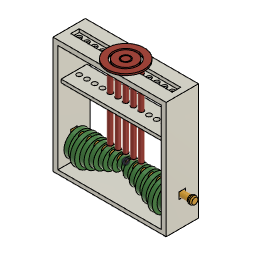
water-drop-mech (Autodesk Fusion 360 design; units mm, degrees)
Autodesk Fusion 360 part; units mm, degrees
note: some values were not read from the file. Set by a fixed rule: which face or edge a step refers to.
sketch "holder body" plane through (0, 0, 0) normal (0, 1, 0) x (1, 0, 0) in component "holder"
  line L0 (107, -220) -> (-68, -220)
  line L1 (-68, -220) -> (-68, -40)
  line L2 (-68, -40) -> (107, -40)
  line L3 (107, -40) -> (107, -220)
  line L4 (107, -220) -> (97, -220)
  line L5 (107, -210) -> (107, -220)
  line L6 (-68, -40) -> (-58, -40)
  line L7 (-68, -50) -> (-68, -40)
  line L8 (97, -210) -> (97, -170)
  line L9 (107, -170) -> (107, -210)
  line L10 (97, -170) -> (-58, -170)
  line L11 (-68, -170) -> (-68, -160)
  line L12 (-58, -160) -> (97, -160)
  line L13 (107, -160) -> (107, -170)
  line L14 (97, -210) -> (-68, -210)
  line L15 (-68, -210) -> (-68, -220)
  line L16 (-68, -220) -> (97, -220)
  line L17 (-68, -50) -> (-68, -210)
  line L18 (-58, -210) -> (-58, -50)
  line L19 (-58, -50) -> (97, -50)
  line L20 (107, -50) -> (107, -40)
  line L21 (107, -40) -> (-58, -40)
  line L22 (107, -170) -> (107, -50)
  line L23 (97, -50) -> (97, -170)
  dimension "d1" = 175
  dimension "d2" = 180
  dimension "d3" = 10
  dimension "d4" = 10
  dimension "d5" = 10
  dimension "d6" = 10
  dimension "d7" = 10
  dimension "d8" = 175
  dimension "d9" = 10
  constraint horizontal L0
  constraint vertical L1
  constraint horizontal L2
  constraint vertical L3
  constraint horizontal L4
  constraint vertical L5
  constraint horizontal L6
  constraint vertical L7
  constraint vertical L8
  constraint vertical L9
  constraint horizontal L10
  constraint vertical L11
  constraint horizontal L12
  constraint vertical L13
  constraint horizontal L14
  constraint vertical L15
  constraint horizontal L16
  constraint vertical L17
  constraint vertical L18
  constraint horizontal L19
  constraint vertical L20
  constraint horizontal L21
  constraint vertical L22
  constraint vertical L23
  constraint coincident L23 L12.end
  constraint coincident L18 L10.end
  constraint coincident L18 L12.start
  measures "d1" distance of L0.start L0.end
  measures "d2" distance of L0.start L2.end
  measures "d3" distance of L0.start L4.end
  measures "d4" distance of L0.start L5.start
  measures "d5" distance of L1.end L6.end
  measures "d6" distance of L1.end L7.start
  measures "d7" distance of L5.start L8.start
  measures "d8" distance of L9.start L11.start
  measures "d9" distance of L9.start L13.start
extrude "Extrude1" add sketch "holder body" against normal blind 50 makes body 1 in component "holder"
sketch "holder top holes" plane through (0, 0, 220) normal (0, 0, 1) x (-1, 0, 0) in component "holder"
  line L0 (-107, 0) -> (68, 0)
  line L1 (68, 0) -> (68, 50)
  line L2 (68, 50) -> (-107, 50)
  line L3 (-107, 50) -> (-107, 0)
  circle A0 centre (-19.5, 25) radius 3.75
  circle A1 centre (-31.5, 25) radius 3.75
  circle A2 centre (-43.5, 25) radius 3.75
  circle A3 centre (-55.5, 25) radius 3.75
  circle A4 centre (-67.5, 25) radius 3.75
  circle A5 centre (-79.5, 25) radius 3.75
  circle A6 centre (-91.5, 25) radius 3.75
  line L4 (-71.25, 25) -> (-75.75, 25)
  line L5 (-83.25, 25) -> (-87.75, 25)
  line L6 (-95.25, 25) -> (-107, 25)
  line L7 (-59.25, 25) -> (-63.75, 25)
  line L8 (-47.25, 25) -> (-51.75, 25)
  line L9 (-35.25, 25) -> (-39.75, 25)
  line L10 (-23.25, 25) -> (-27.75, 25)
  line L11 (-19.5, 0) -> (-19.5, 21.25)
  line L12 (-19.5, 28.75) -> (-19.5, 50)
  circle A7 centre (-7.5, 25) radius 3.75
  circle A8 centre (4.5, 25) radius 3.75
  circle A9 centre (16.5, 25) radius 3.75
  circle A10 centre (28.5, 25) radius 3.75
  circle A11 centre (40.5, 25) radius 3.75
  circle A12 centre (52.5, 25) radius 3.75
  line L13 (52.5, 25) -> (59, 25)
  line L14 (59, 25) -> (59, 18.5)
  line L15 (-91.5, 25) -> (-98, 25)
  line L16 (-98, 25) -> (-98, 31.5)
  line L17 (-98, 31.5) -> (59, 31.5)
  line L18 (59, 31.5) -> (59, 18.5)
  line L19 (59, 18.5) -> (-98, 18.5)
  line L20 (-98, 18.5) -> (-98, 31.5)
  dimension "d12" = 7.5
  dimension "d15" = 72
  dimension "d16" = 0
  dimension "d19" = 6.5
  dimension "d20" = 6.5
  dimension "d21" = 6.5
  constraint midpoint L3 L6.end
  constraint midpoint L0 L11.start
  constraint perpendicular L0 L11
  constraint coincident A4 L7.end
  constraint coincident A4 L4.start
  constraint coincident A5 L4.end
  constraint coincident A5 L5.start
  constraint collinear L4 L5
  constraint coincident A6 L5.end
  constraint coincident A6 L6.start
  constraint collinear L5 L6
  constraint coincident A3 L8.end
  constraint coincident A3 L7.start
  constraint coincident A2 L9.end
  constraint coincident A2 L8.start
  constraint coincident A1 L10.end
  constraint coincident A1 L9.start
  constraint coincident A0 L10.start
  constraint coincident A0 L11.end
  constraint coincident A0 L12.start
  constraint collinear L11 L12
  constraint symmetric A1 L11 A7
  constraint symmetric A2 L11 A8
  constraint symmetric A3 L11 A9
  constraint symmetric A4 L11 A10
  constraint symmetric A5 L11 A11
  constraint symmetric A6 L11 A12
  constraint coincident A12.centre L13.start
  constraint horizontal L13
  constraint perpendicular L13 L14
  constraint coincident A6.centre L15.start
  constraint parallel L6 L15
  constraint perpendicular L6 L16
  constraint horizontal L17
  constraint vertical L18
  constraint horizontal L19
  constraint vertical L20
  measures "d12" diameter of A0
  measures "d19" distance of L13.end L14.end
  measures "d20" distance of A6.centre L15.end
  measures "d21" distance of L15.end L16.end
extrude "Extrude3" cut sketch "holder top holes" against normal blind 5 contours A0 A1 A2 A3 A4 A5 A6 L4 L5 L6 L7 L8 L9 L10 L11 L15 L19 L20 | A0 L11 L12 L14 L17 L18 L19 | A0 A1 A2 A3 A4 A5 A6 L4 L5 L6 L7 L8 L9 L10 L12 L15 L16 L17 L20 bodies 1 in component "holder"
extrude "Extrude2" cut sketch "holder top holes" against normal blind 44 contours A0 | A6 | A1 | A5 | A2 | A4 | A3 | A7 | A8 | A9 | A10 | A11 | A12 bodies 1 in component "holder"
move_face "OffsetFaces1" offset -0.03 13 faces at (-44.2314, -24.6266, 213.3333) (-56.2314, -24.6266, 213.3333) (-32.2314, -24.6266, 213.3333) (-20.2314, -24.6266, 213.3333) (-8.2314, -24.6266, 213.3333) (3.7686, -24.6266, 213.3333) (15.7686, -25.3734, 213.3333) (27.7686, -25.3734, 213.3333) (39.7686, -25.3734, 213.3333) (51.7686, -25.3734, 213.3333) (63.7686, -25.3734, 213.3333) (75.7686, -25.3734, 213.3333) (87.7686, -25.3734, 213.3333) on bodies 1 in component "holder"
sketch "holder side details" plane through (107, 0, 0) normal (1, 0, 0) x (0, 1, 0) in component "holder"
  line L0 (0, 40) -> (0, 220)
  line L1 (-50, 220) -> (-50, 40)
  line L2 (-50, 40) -> (0, 40)
  line L3 (-50, 40) -> (0, 40)
  line L4 (0, 40) -> (0, 220)
  line L5 (0, 220) -> (-50, 220)
  line L6 (-50, 220) -> (-50, 40)
  line L7 (-25, 40) -> (-25, 220)
  line L8 (-25, 220) -> (-25, 160)
  line L9 (-25, 40) -> (-25, 85)
  line L10 (-20, 80) -> (-30, 80)
  line L11 (-30, 80) -> (-30, 90)
  line L12 (-30, 90) -> (-20, 90)
  line L13 (-20, 90) -> (-20, 80)
  line L14 (-20, 80) -> (-30, 90) construction
  line L15 (-30, 80) -> (-20, 90) construction
  line L16 (-5, 155) -> (-45, 155)
  line L17 (-45, 155) -> (-45, 165)
  line L18 (-45, 165) -> (-5, 165)
  line L19 (-5, 165) -> (-5, 155)
  line L20 (-5, 155) -> (-45, 165) construction
  line L21 (-45, 155) -> (-5, 165) construction
  line L22 (0, 220) -> (-50, 220)
  point P0 (-25, 85)
  point P1 (-25, 160)
  dimension "d26" = 60
  dimension "d27" = 45
  constraint horizontal L3
  constraint vertical L4
  constraint horizontal L5
  constraint vertical L6
  constraint coincident L0.end L4.end
  constraint coincident L1.end L2.start
  constraint midpoint L3 L7.start
  constraint midpoint L5 L7.end
  constraint perpendicular L5 L8
  constraint perpendicular L3 L9
  constraint horizontal L10
  constraint perpendicular L10 L11
  constraint parallel L10 L12
  constraint parallel L11 L13
  constraint coincident L14 P0
  constraint coincident L15 P0
  constraint coincident P0 L9.end
  constraint horizontal L16
  constraint perpendicular L16 L17
  constraint parallel L16 L18
  constraint parallel L17 L19
  constraint coincident L20 P1
  constraint coincident L21 P1
  constraint coincident P1 L8.end
  measures "d26" distance of L7.end P1
  measures "d27" distance of L7.start P0
extrude "Extrude4" cut sketch "holder side details" against normal blind 260 contours L7 L9 L10 L11 L12 | L7 L9 L10 L12 L13 bodies 1 in component "holder"
extrude "Extrude5" add sketch "holder side details" against normal blind 165 contours L7 L8 L16 L18 L19 | L7 L8 L16 L17 L18 bodies 1 in component "holder"
extrude "Extrude6" cut sketch "holder top holes" against normal blind 125 contours A0 | A6 | A1 | A5 | A2 | A4 | A3 | A7 | A8 | A9 | A10 | A11 | A12 bodies 1 in component "holder"
move_face "OffsetFaces2" offset -0.03 13 faces at (75.7686, -24.6266, 161.6667) (87.7686, -24.6266, 161.6667) (63.7686, -24.6266, 161.6667) (51.7686, -24.6266, 161.6667) (39.7686, -24.6266, 161.6667) (27.7686, -24.6266, 161.6667) (15.7686, -24.6266, 161.6667) (3.7686, -24.6266, 161.6667) (-8.2314, -24.6266, 161.6667) (-20.2314, -24.6266, 161.6667) (-32.2314, -24.6266, 161.6667) (-44.2314, -24.6266, 161.6667) (-56.2314, -24.6266, 161.6667) on bodies 1 in component "holder"
extrude "Extrude7" cut 1 faces at (97, -23.3333, 133.3333) along direction (1, 0, 0) blind 2.5 on bodies 1 bodies 1 in component "holder"
extrude "Extrude8" cut 1 faces at (-58, -23.3333, 133.3333) along direction (-1, 0, 0) blind 2.5 on bodies 1 bodies 1 in component "holder"
sketch "support rod" plane through (0, 0, 0) normal (1, 0, 0) x (0, 1, 0) in component "support rod"
  circle A0 centre (0, 0) radius 5
  dimension "d40" = 10
  constraint coincident A0.centre origin
  measures "d40" diameter of A0
extrude "Extrude1'" add sketch "support rod" along normal blind 100 and the other way blind 100 separate body makes body 2 in component "support rod"
move_face "OffsetFaces1'" offset -0.2 2 faces at (33.3333, 4.9752, -0.4978) (-33.3333, 4.9752, -0.4978) on bodies 2 in component "support rod"
extrude "Extrude2'" add 1 faces at (100, 1.1814, 0.0314) along direction (1, 0, 0) blind 2.5 draft 25 on bodies 2 bodies 2 in component "support rod"
extrude "Extrude3'" add 1 faces at (102.5, 1.4577, 1.3526) along direction (1, 0, 0) blind 2 on bodies 2 bodies 2 in component "support rod"
extrude "Extrude4'" add 1 faces at (104.5, 1.4577, 1.3526) along direction (1, 0, 0) blind 2.5 draft -25 on bodies 2 bodies 2 in component "support rod"
sketch "support circle 1" plane through (0, 0, 0) normal (1, 0, 0) x (0, 1, 0) in component "support circle 1"
  circle A0 centre (30, 20) radius 10
  circle A1 centre (30, 22) radius 5
  dimension "d52" = 10
  measures "d52" diameter of A1
extrude "Extrude1''" add sketch "support circle 1" against normal blind 7 separate body makes body 3 in component "support circle 1"
sketch "support circle 2" plane through (0, 0, 0) normal (1, 0, 0) x (0, 1, 0) in component "support circle 2"
  circle A0 centre (0, 0) radius 12.5
  circle A1 centre (0, 5) radius 5
  dimension "d55" = 25
  constraint coincident A0.centre origin
  constraint coincident A0.centre A1
  measures "d55" diameter of A0
extrude "Extrude1'''" add sketch "support circle 2" along normal blind 7 separate body makes body 4 in component "support circle 2"
sketch "support circle 3" plane through (0, 0, 0) normal (1, 0, 0) x (0, 1, 0) in component "support circle 3"
  circle A0 centre (0, 0) radius 15
  circle A1 centre (0, 7.5) radius 5
  constraint coincident A0.centre origin
extrude "Extrude1''''" add sketch "support circle 3" against normal blind 7 separate body makes body 5 in component "support circle 3"
sketch "support circle 4" plane through (0, 0, 0) normal (1, 0, 0) x (0, 1, 0) in component "support circle 4"
  circle A0 centre (0, 0) radius 17.5
  circle A1 centre (0, 10) radius 5
  dimension "d60" = 35
  constraint coincident A0.centre origin
  measures "d60" diameter of A0
extrude "Extrude1'''''" add sketch "support circle 4" along normal blind 7 separate body makes body 6 in component "support circle 4"
sketch "support circle 5" plane through (0, 0, 0) normal (1, 0, 0) x (0, 1, 0) in component "support circle 5"
  circle A0 centre (0, -2.5) radius 20
  circle A1 centre (0, 10) radius 5
extrude "Extrude1''''''" add sketch "support circle 5" along normal blind 7 separate body makes body 7 in component "support circle 5"
sketch "support circle 6" plane through (0, 0, 0) normal (1, 0, 0) x (0, 1, 0) in component "support circle 6"
  circle A0 centre (0, -5) radius 22.5
  circle A1 centre (0, 10) radius 5
  line L0 (0, 0) -> (0, -5)
  dimension "d65" = 45
  dimension "d227" = 5
  constraint coincident L0.start origin
  constraint vertical L0
  measures "d65" diameter of A0
  measures "d227" distance of L0.start A0.centre
extrude "Extrude1'''''''" add sketch "support circle 6" along normal blind 7 separate body makes body 8 in component "support circle 6"
sketch "top circle 1" plane through (0, 0, 0) normal (0, 0, 1) x (1, 0, 0) in component "top circle 1"
  circle A0 centre (0, 50) radius 3.75
  circle A1 centre (0, 50) radius 5.75
  dimension "d68" = 7.5
  dimension "d69" = 11.5
  constraint concentric A0 A1
  measures "d68" diameter of A0
  measures "d69" diameter of A1
extrude "Extrude1''''''''" add sketch "top circle 1" along normal blind 2.5 separate body contours A0 | A1 makes body 9 in component "top circle 1"
extrude "Extrude2''" add sketch "holder top holes" against normal blind 127 contours A0 sketch seen with x (1, 0, 0) y (0, 1, 0) z (0, 0, 1) at (-19.5, 75, -220) bodies 9 in component "top circle 1"
sketch "top circle 2" plane through (0, 0, 0) normal (0, 0, 1) x (1, 0, 0) in component "top circle 2"
  circle A0 centre (0, 100) radius 3.75
  line L0 (0, 100) -> (8.25, 100)
  circle A1 centre (12, 100) radius 3.75
  circle A2 centre (0, 100) radius 16.75
  circle A3 centre (0, 100) radius 7.25
  line L1 (0, 100) -> (0, 107.25)
  circle A4 centre (-12, 100) radius 3.75
  dimension "d74" = 7.5
  dimension "d75" = 8.25
  dimension "d76" = 7.5
  dimension "d77" = 33.5
  dimension "d78" = 14.5
  constraint coincident A0.centre L0.start
  constraint horizontal L0
  constraint coincident L0.end A1
  constraint concentric A0 A2
  constraint concentric A0 A3
  constraint coincident A3 L1.end
  constraint perpendicular L0 L1
  constraint symmetric A1 L1 A4
  measures "d74" diameter of A0
  measures "d75" distance of A0.centre L0.end
  measures "d76" diameter of A1
  measures "d77" diameter of A2
  measures "d78" diameter of A3
extrude "Extrude1'''''''''" add sketch "top circle 2" along normal blind 2.5 separate body contours A1 | A2 | A4 makes body 10 in component "top circle 2"
extrude "Extrude2'''" add sketch "top circle 2" against normal blind 127.5 contours A1 | A4 bodies 10 in component "top circle 2"
sketch "top circle 3" plane through (0, 0, 0) normal (0, 0, 1) x (1, 0, 0) in component "top circle 3"
  circle A0 centre (0, 50) radius 3.75
  line L0 (0, 50) -> (12, 50)
  circle A1 centre (12, 50) radius 3.75
  line L1 (12, 50) -> (24, 50)
  circle A2 centre (24, 50) radius 3.75
  circle A3 centre (0, 50) radius 28.75
  circle A4 centre (0, 50) radius 19.25
  line L2 (0, 50) -> (0, 46.25)
  circle A5 centre (-24, 50) radius 3.75
  dimension "d83" = 7.5
  dimension "d84" = 12
  dimension "d85" = 7.5
  dimension "d86" = 12
  dimension "d87" = 7.5
  dimension "d88" = 57.5
  dimension "d89" = 38.5
  constraint coincident A0.centre L0.start
  constraint horizontal L0
  constraint coincident L0.end A1.centre
  constraint parallel L0 L1
  constraint coincident L1.end A2.centre
  constraint concentric A0 A3
  constraint concentric A3 A4
  constraint coincident A0 L2.end
  constraint perpendicular L0 L2
  constraint symmetric A2 L2 A5
  measures "d83" diameter of A0
  measures "d84" distance of A0.centre L0.end
  measures "d85" diameter of A1
  measures "d86" distance of L0.end L1.end
  measures "d87" diameter of A2
  measures "d88" diameter of A3
  measures "d89" diameter of A4
extrude "Extrude1''''''''''" add sketch "top circle 3" along normal blind 2.5 separate body contours A2 | A3 | A5 makes body 11 in component "top circle 3"
extrude "Extrude2''''" add sketch "top circle 3" against normal blind 127.5 contours A2 | A5 bodies 11 in component "top circle 3"
sketch "top circle 4" plane through (0, 0, 0) normal (0, 0, 1) x (1, 0, 0) in component "top circle 4"
  circle A0 centre (0, 100) radius 3.75
  line L0 (0, 100) -> (12, 100)
  line L1 (12, 100) -> (24, 100)
  line L2 (24, 100) -> (36, 100)
  circle A1 centre (36, 100) radius 3.75
  circle A2 centre (0, 100) radius 31.25
  circle A3 centre (0, 100) radius 40.75
  line L3 (0, 100) -> (0, 96.25)
  circle A4 centre (-36, 100) radius 3.75
  dimension "d94" = 7.5
  dimension "d95" = 12
  dimension "d96" = 12
  dimension "d97" = 12
  dimension "d98" = 7.5
  dimension "d99" = 62.5
  dimension "d100" = 81.5
  constraint coincident A0.centre L0.start
  constraint horizontal L0
  constraint parallel L0 L1
  constraint parallel L1 L2
  constraint coincident L2.end A1.centre
  constraint concentric A0 A2
  constraint concentric A0 A3
  constraint coincident A0 L3.end
  constraint perpendicular L0 L3
  constraint symmetric A1 L3 A4
  measures "d94" diameter of A0
  measures "d95" distance of A0.centre L0.end
  measures "d96" distance of L0.end L1.end
  measures "d97" distance of L1.end L2.end
  measures "d98" diameter of A1
  measures "d99" diameter of A2
  measures "d100" diameter of A3
extrude "Extrude1'''''''''''" add sketch "top circle 4" along normal blind 2.5 separate body contours A1 | A3 | A4 makes body 12 in component "top circle 4"
extrude "Extrude2'''''" add sketch "top circle 4" against normal blind 127.5 contours A1 | A4 bodies 12 in component "top circle 4"
sketch "top circle 6" plane through (0, 0, 0) normal (0, 0, 1) x (1, 0, 0) in component "top circle 6"
  circle A0 centre (0, 100) radius 3.75
  line L0 (0, 100) -> (60, 100)
  circle A1 centre (60, 100) radius 3.75
  line L1 (0, 100) -> (0, 103.75)
  circle A2 centre (-60, 100) radius 3.75
  circle A3 centre (0, 100) radius 55.25
  circle A4 centre (0, 100) radius 64.75
  dimension "d105" = 7.5
  dimension "d106" = 60
  dimension "d107" = 7.5
  dimension "d108" = 110.5
  dimension "d109" = 129.5
  constraint coincident A0.centre L0.start
  constraint horizontal L0
  constraint coincident L0.end A1.centre
  constraint coincident A0 L1.end
  constraint perpendicular L0 L1
  constraint symmetric A1 L1 A2
  constraint concentric A0 A3
  constraint concentric A3 A4
  measures "d105" diameter of A0
  measures "d106" distance of A0.centre L0.end
  measures "d107" diameter of A1
  measures "d108" diameter of A3
  measures "d109" diameter of A4
extrude "Extrude1''''''''''''" add sketch "top circle 6" along normal blind 2.5 separate body contours A1 | A2 | A4 makes body 13 in component "top circle 6"
extrude "Extrude2''''''" add sketch "top circle 6" against normal blind 122.5 contours A1 | A2 bodies 13 in component "top circle 6"
sketch "top circle 5" plane through (0, 0, 0) normal (0, 0, 1) x (1, 0, 0) in component "top circle 5"
  line L0 (0, 150) -> (48, 150)
  circle A0 centre (48, 150) radius 3.75
  circle A1 centre (0, 150) radius 43.25
  circle A2 centre (0, 150) radius 52.75
  line L1 (0, 150) -> (0, 193.25)
  circle A3 centre (-48, 150) radius 3.75
  dimension "d114" = 48
  dimension "d115" = 7.5
  dimension "d116" = 86.5
  dimension "d117" = 105.5
  constraint horizontal L0
  constraint coincident L0.end A0.centre
  constraint coincident L0.start A1.centre
  constraint concentric A1 A2
  constraint coincident A1 L1.end
  constraint perpendicular L0 L1
  constraint symmetric A0 L1 A3
  measures "d114" distance of L0.start L0.end
  measures "d115" diameter of A0
  measures "d116" diameter of A1
  measures "d117" diameter of A2
extrude "Extrude1'''''''''''''" add sketch "top circle 5" along normal blind 2.5 separate body contours A0 | A2 | A3 makes body 14 in component "top circle 5"
extrude "Extrude2'''''''" add sketch "top circle 5" against normal blind 125 contours A0 | A3 bodies 14 in component "top circle 5"
sketch "top circle 7" plane through (0, 0, 0) normal (0, 0, 1) x (1, 0, 0) in component "top circle 7"
  line L0 (0, 150) -> (72, 150)
  circle A0 centre (72, 150) radius 3.75
  line L1 (0, 150) -> (0, 160)
  circle A1 centre (-72, 150) radius 3.75
  circle A2 centre (0, 150) radius 67.25
  circle A3 centre (0, 150) radius 76.75
  dimension "d122" = 72
  dimension "d123" = 7.5
  dimension "d124" = 134.5
  dimension "d125" = 153.5
  constraint horizontal L0
  constraint coincident L0.end A0.centre
  constraint perpendicular L0 L1
  constraint symmetric A0 L1 A1
  constraint coincident L0.start L1.start
  constraint concentric A2 A3
  measures "d122" distance of L0.start L0.end
  measures "d123" diameter of A0
  measures "d124" diameter of A2
  measures "d125" diameter of A3
extrude "Extrude1''''''''''''''" add sketch "top circle 7" along normal blind 2.5 separate body contours A0 | A1 | A3 makes body 15 in component "top circle 7"
extrude "Extrude2''''''''" add sketch "top circle 7" against normal blind 125 contours A0 | A1 bodies 15 in component "top circle 7"
fillet "Fillet1" radius 3.75 1 edges at (3.4962, 48.6439, -127) on bodies 9 in component "top circle 1"
extrude "Extrude9" cut 1 faces at (-7.1667, -33.3333, 50) along direction (0, 0, -1) blind 2.5 on bodies 1 bodies 1 in component "holder"
extrude "Extrude10" cut 1 faces at (19.5942, -42.9231, 210) along direction (0, 0, 1) blind 2.5 on bodies 1 bodies 1 in component "holder"
extrude "Extrude11" cut 1 faces at (23.4058, -39.5898, 155) along direction (0, 0, 1) blind 5 on bodies 1 bodies 1 in component "holder"
extrude "Extrude12" cut 1 faces at (-7.1667, -33.3333, 47.5) along direction (0, 0, -1) blind 1.5 on bodies 1 bodies 1 in component "holder"
fillet "Fillet1'" radius 3.5 1 edges at (-15.4962, 101.3561, -127.5) on bodies 10 in component "top circle 2"
fillet "Fillet2" radius 3.5 1 edges at (8.5038, 101.3561, -127.5) on bodies 10 in component "top circle 2"
fillet "Fillet1''" radius 3.5 1 edges at (20.5038, 51.3561, -127.5) on bodies 11 in component "top circle 3"
fillet "Fillet2'" radius 3.5 1 edges at (-27.4962, 51.3561, -127.5) on bodies 11 in component "top circle 3"
component "holder" placed x (1, 0, 0) y (0, 1, 0) z (0, 0, 1) at (0, 0, 0)
component "support rod" placed x (1, 0, 0) y (0, 1, 0) z (0, 0, 1) at (19.5, -25, 85)
component "support circle 1" placed x (1, 0, 0) y (0, 1, 0) z (0, 0, 1) at (23, -55, 63)
component "support circle 2" placed x (1, 0, 0) y (0, 1, 0) z (0, 0, 1) at (4, -25, 80)
component "support circle 2" placed x (1, 0, 0) y (0, 1, 0) z (0, 0, 1) at (28, -25, 80)
component "support circle 3" placed x (1, 0, 0) y (0, 1, 0) z (0, 0, 1) at (47, -25, 77.5)
component "support circle 3" placed x (1, 0, 0) y (0, 1, 0) z (0, 0, 1) at (-1, -25, 77.5)
component "support circle 4" placed x (1, 0, 0) y (0, 1, 0) z (0, 0, 1) at (52, -25, 75)
component "support circle 4" placed x (1, 0, 0) y (0, 1, 0) z (0, 0, 1) at (-20, -25, 75)
component "support circle 5" placed x (1, 0, 0) y (0, 1, 0) z (0, 0, 1) at (64, -25, 75)
component "support circle 5" placed x (1, 0, 0) y (0, 1, 0) z (0, 0, 1) at (-32, -25, 75)
component "support circle 6" placed x (1, 0, 0) y (0, 1, 0) z (0, 0, 1) at (76, -25, 75)
component "support circle 6" placed x (1, 0, 0) y (0, 1, 0) z (0, 0, 1) at (-44, -25, 75)
component "support circle 5" placed x (1, 0, 0) y (0, 1, 0) z (0, 0, 1) at (88, -25, 75)
component "support circle 5" placed x (1, 0, 0) y (0, 1, 0) z (0, 0, 1) at (-56, -25, 75)
component "top circle 1" placed x (1, 0, 0) y (0, 1, 0) z (0, 0, 1) at (19.5, -75, 220)
component "top circle 2" placed x (1, 0, 0) y (0, 1, 0) z (0, 0, 1) at (19.5, -125, 220)
component "top circle 3" placed x (1, 0, 0) y (0, 1, 0) z (0, 0, 1) at (19.5, -75, 220)
component "top circle 4" placed x (1, 0, 0) y (0, 1, 0) z (0, 0, 1) at (19.5, -125, 220)
component "top circle 6" placed x (1, 0, 0) y (0, 1, 0) z (0, 0, 1) at (19.5, -125, 220)
component "top circle 5" placed x (1, 0, 0) y (0, 1, 0) z (0, 0, 1) at (19.5, -175, 220)
component "top circle 7" placed x (1, 0, 0) y (0, 1, 0) z (0, 0, 1) at (19.5, -175, 220)
component "support circles" placed x (1, 0, 0) y (0, 1, 0) z (0, 0, 1) at (0, 0, 0)
equation "d69 = 7.5 mm + ( 2 * 2 ) * 1 mm"
equation "d75 = 3.75 mm + 4.5 mm"
equation "d77 = 31.5 mm + 2 mm"
equation "d84 = 7.5 mm + 4.5 mm"
equation "d86 = 7.5 mm + 4.5 mm"
equation "d88 = 55.5 mm + 2 mm"
equation "d89 = 40.5 mm - 2 mm"
equation "d95 = 7.5 mm + 4.5 mm"
equation "d99 = 64.5 mm - 2 mm"
equation "d106 = ( 12 * 5 ) * 1 mm"
equation "d114 = ( 12 * 4 ) * 1 mm"
equation "d122 = ( 12 * 6 ) * 1 mm"
named bodies: "support circle 1", "support circle 2", "support circle 3", "support circle 4", "support circle 5", "support circle 6", "top circle 1", "top circle 2", "top circle 3", "top circle 4", "top circle 6", "top circle 5", "top circle 7"
